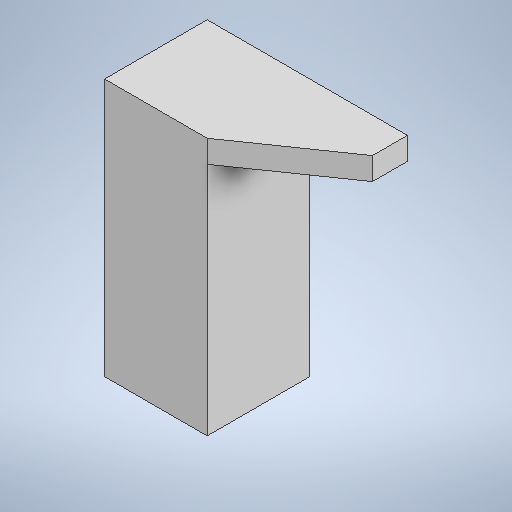
# Autodesk Inventor part: Pata1
Saved by Autodesk Inventor 2025 (Build 290162000, 162)
## iProperties
Created: 2026-09-16
Part Number: Pata1
Material: Genérico
Document SubType Name: Modeling
Designer: ASUS
Density: 1 g/cm^3
Appearance: Valor por defecto
Author: ASUS
Autodesk Inventor part; units mm, degrees
ref_plane "YZ Plane" through (0, 0, 0) normal (1, 0, 0) x (0, 1, 0)
ref_plane "XZ Plane" through (0, 0, 0) normal (0, 1, 0) x (-1, 0, 0)
ref_plane "XY Plane" through (0, 0, 0) normal (0, 0, 1) x (1, 0, 0)
sketch "Boceto1" plane through (0, 0, 0) normal (0, 1, 0) x (-1, 0, 0)
  line L0 (20.5, -20.5) -> (-20.5, -20.5)
  line L1 (-20.5, -20.5) -> (-20.5, 20.5)
  line L2 (-20.5, 20.5) -> (20.5, 20.5)
  line L3 (20.5, 20.5) -> (20.5, -20.5)
  point P0 (0, 0)
  point P1 (0, -20.5)
  point P2 (-20.5, 0)
  dimension "d0" = 41
  dimension "d1" = 41
  constraints: 8 end point, 2 midpoint, 2 parallel, 1 horizontal, 1 horizontal alignment, 1 perpendicular, 1 vertical alignment
  measures "d0" distance of L1.end L2.end
  measures "d1" distance of L0.end L1.end
extrude "Extrusión1" add sketch "Boceto1" along normal blind 94
sketch "Boceto2" plane through (0, 94, 0) normal (0, 1, 0) x (1, 0, 0)
  line L0 (20.5, 20.5) -> (-20.5, 20.5) projected
  line L1 (-20.5, 20.5) -> (59.5, 20.5)
  line L2 (59.5, 20.5) -> (59.5, 6.5)
  line L3 (-20.5, -20.5) -> (20.5, -20.5) projected
  line L4 (59.5, 6.5) -> (20.5, -20.5)
  line L5 (20.5, -20.5) -> (20.5, 20.5) projected
  line L6 (50.8333, 0.5) -> (20.5, 0.5)
  line L7 (22.5, 18.5) -> (57.5, 18.5)
  line L8 (57.5, 18.5) -> (57.5, 7.5479)
  line L9 (57.5, 7.5479) -> (50.2086, 2.5)
  line L10 (22.5, 18.5) -> (22.5, 2.5)
  line L11 (22.5, 2.5) -> (50.2086, 2.5)
  line L12 (22.5, 0.5) -> (22.5, -16.6829)
  line L13 (22.5, -16.6829) -> (47.3197, 0.5)
  point P0 (0, 0)
  point P1 (36.3543, 2.5)
  dimension "d4" = 80
  dimension "d5" = 14
  dimension "d9" = 2
  dimension "d10" = 2
  dimension "d11" = 2
  dimension "d12" = 2
  dimension "d13" = 2
  dimension "d20" = 5.0479
  constraints: 22 end point, 7 point on line, 2 horizontal, 2 perpendicular, 1 collinear, 1 midpoint, 1 parallel, 1 vertical
  measures "d4" distance of L0.end L1.end
  measures "d5" distance of L1.end L2.end
  measures "d9" distance between parallel lines of L1 L7
  measures "d10" distance between parallel lines of L8 L2
  measures "d11" distance between parallel lines of L4 L9
  measures "d12" distance between parallel lines of L5 L10
  measures "d13" distance from line of L6 point (36.354, 2.5)
  measures "d20" vertical distance of L8.end L9.end
extrude "Extrusión2" add sketch "Boceto2" along normal blind 8 contours L1 L2 L4 L6 L5 | L6 L12 L13 L4 L5
sketch "Boceto3" plane through (0, 94, 0) normal (0, 1, 0) x (1, 0, 0)
  line L0 (-20.5, 20.5) -> (-20.5, -20.5) projected
  line L1 (20.5, -20.5) -> (59.5, 6.5) projected
  line L2 (-20.5, 20.5) -> (20.5, 20.5)
  line L3 (20.5, 20.5) -> (20.5, -20.5)
  line L4 (20.5, -20.5) -> (-20.5, -20.5)
  line L5 (-20.5, -20.5) -> (-20.5, 20.5)
  point P0 (0, 0)
  constraints: 8 end point, 2 parallel, 1 horizontal, 1 perpendicular
extrude "Extrusión3" add sketch "Boceto3" along normal blind 8
sketch "Boceto4" plane through (0, 102, 0) normal (0, 1, 0) x (1, 0, 0)
  point P0 (0, 0)
sketch "Boceto6" plane through (0, 102, 0) normal (0, 1, 0) x (1, 0, 0)
  line L0 (-20.5, 20.5) -> (-20.5, -20.5) projected
  line L1 (59.5, 6.5) -> (59.5, 20.5) projected
  line L2 (-20.5, 20.5) -> (59.5, 20.5)
  line L3 (59.5, 20.5) -> (59.5, 6.5)
  line L4 (20.5, -20.5) -> (59.5, 6.5) projected
  line L5 (59.5, 6.5) -> (20.5, -20.5)
  line L6 (20.5, -20.5) -> (-20.5, -20.5)
  line L7 (-20.5, -20.5) -> (-20.5, 20.5)
  point P0 (0, 0)
  constraints: 10 end point, 3 perpendicular, 1 collinear, 1 parallel
extrude "Extrusión5" add sketch "Boceto6" along normal blind 1
